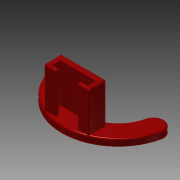
# Autodesk Inventor part: Camerahouder
Saved by Autodesk Inventor 2015 (Build 190159000, 159)
## iProperties
Created: 2016-04-29
Part Number: Camerahouder
Material: Generic
Document SubType Name: Modeling
Designer: david
Density: 1 g/cm^3
Appearance: Red
Author: david
Autodesk Inventor part; units mm, degrees
ref_plane "YZ Plane" through (0, 0, 0) normal (1, 0, 0) x (0, 1, 0)
ref_plane "XZ Plane" through (0, 0, 0) normal (0, 1, 0) x (-1, 0, 0)
ref_plane "XY Plane" through (0, 0, 0) normal (0, 0, 1) x (1, 0, 0)
sketch "Sketch1" plane through (0, 0, 0) normal (0, 0, 1) x (1, 0, 0)
  circle A0 centre (0, 0) radius 27.5
  circle A1 centre (0, 0) radius 42.5
  line L0 (27.5, 0) -> (42.5, 0)
  line L1 (-27.5, 0) -> (-42.5, 0)
  dimension "d0" = 55
  dimension "d1" = 85
  constraints: 4 end point, 4 point on circle, 2 centre point, 2 coincident, 2 point on line, 1 horizontal
  measures "d0" diameter of A0
  measures "d1" diameter of A1
extrude "Extrusion1" add sketch "Sketch1" along normal blind 5 contours L0 A1 L1 A0 picked at (1.1049, -37.278)
fillet "Fillet1" radius 7.5 4 edges at (-27.5, 0, 2.5) (-42.5, 0, 2.5) (27.5, 0, 2.5) (42.5, 0, 2.5)
sketch "Sketch2" plane through (0, 0, 5) normal (0, 0, 1) x (1, 0, 0)
  line L0 (15, -30) -> (-15, -30)
  line L1 (-15, -30) -> (-15, -38.9796)
  line L2 (-15, -38.9796) -> (15, -38.9796)
  line L3 (15, -38.9796) -> (15, -30)
  line L4 (15, -30) -> (-15, -38.9796) construction
  line L5 (-15, -30) -> (15, -38.9796) construction
  point P0 (0, 0)
  point P1 (0, -34.4898)
  dimension "d5" = 30
  dimension "d6" = 30
  constraints: 12 end point, 2 midpoint, 2 parallel, 1 horizontal, 1 perpendicular
  measures "d5" distance of L1.end L2.end
  measures "d6" distance from line of point (0, 0) L0
extrude "Extrusion2" add sketch "Sketch2" along normal blind 30
sketch "Sketch3" plane through (0, 0, 35) normal (0, 0, 1) x (1, 0, 0)
  line L0 (-8, -38.9796) -> (8, -38.9796)
  line L1 (8, -38.9796) -> (8, -35.9796)
  line L2 (8, -35.9796) -> (-8, -35.9796)
  line L3 (-8, -35.9796) -> (-8, -38.9796)
  line L4 (-8, -38.9796) -> (8, -35.9796) construction
  line L5 (8, -38.9796) -> (-8, -35.9796) construction
  line L6 (-15, -38.9796) -> (15, -38.9796) projected
  line L7 (-13, -27.9796) -> (13, -27.9796)
  line L8 (13, -27.9796) -> (13, -35.9796)
  line L9 (13, -35.9796) -> (-13, -35.9796)
  line L10 (-13, -35.9796) -> (-13, -27.9796)
  line L11 (-13, -27.9796) -> (13, -35.9796) construction
  line L12 (13, -27.9796) -> (-13, -35.9796) construction
  point P0 (0, 0)
  point P1 (0, -37.4796)
  point P2 (0, -31.9796)
  dimension "d9" = 16
  dimension "d10" = 3
  dimension "d11" = 0
  dimension "d12" = 26
  dimension "d24" = 8
  constraints: 24 end point, 4 midpoint, 4 parallel, 2 horizontal, 2 perpendicular
  measures "d9" distance of L2.end L1.end
  measures "d10" distance of L2.end L0.start
  measures "d11" distance from line of L6 L0.start
  measures "d12" distance of L8.end L9.end
  measures "d24" distance between parallel lines of L7 L2
extrude "Extrusion3" cut sketch "Sketch3" against normal blind 30
sketch "Sketch4" plane through (-15, -30, 5) normal (0, 1, 0) x (1, 0, 0)
  line L0 (-26.5128, 0) -> (56.5128, 0) projected
  line L1 (30, -30) -> (0, -30)
  line L2 (0, -30) -> (0, 0)
  line L3 (0, 0) -> (30, 0)
  line L4 (30, 0) -> (30, -30)
  line L5 (30, 0) -> (0, 0)
  line L6 (0, 0) -> (0, 5)
  line L7 (0, 5) -> (30, 5)
  line L8 (30, 5) -> (30, 0)
  point P0 (15, 5)
  dimension "d15" = 30
  dimension "d18" = 30
  dimension "d19" = 5
  constraints: 16 end point, 4 parallel, 2 horizontal, 2 perpendicular, 1 point on line
  measures "d15" distance of L2.end L3.end
  measures "d18" distance of L6.end L7.end
  measures "d19" distance between parallel lines of L0 L7
extrude "Extrusion4" add sketch "Sketch4" along normal blind 4 contours L0 L4 L1 L2
sketch "Sketch5" plane through (-15, -38.9796, 5) normal (-1, 0, 0) x (0, 0, 1)
  line L0 (30, 12.9796) -> (0, 12.9796)
  line L1 (0, 12.9796) -> (0, 0)
  line L2 (0, 0) -> (30, 0)
  line L3 (30, 0) -> (30, 12.9796)
  point P0 (-5, 38.9796)
  constraints: 8 end point, 2 parallel, 1 horizontal, 1 perpendicular
extrude "Extrusion5" add sketch "Sketch5" along normal blind 2
sketch "Sketch6" plane through (15, -38.9796, 35) normal (1, 0, 0) x (0, 0, -1)
  line L0 (0, 0) -> (30, 0)
  line L1 (30, 0) -> (30, 12.9796)
  line L2 (30, 12.9796) -> (0, 12.9796)
  line L3 (0, 12.9796) -> (0, 0)
  point P0 (35, 38.9796)
  constraints: 8 end point, 2 parallel, 1 horizontal, 1 perpendicular
extrude "Extrusion6" add sketch "Sketch6" along normal blind 2
fillet "Fillet2" radius 1 10 edges at (17, -38.9796, 20) (8, -38.9796, 20) (-8, -38.9796, 20) (-8, -35.9796, 20) (-17, -38.9796, 20) (17, -26, 20) (-17, -26, 20) (-17, -32.4898, 35) (-12.5, -38.9796, 35) (-13, -32.9898, 35)
fillet "Fillet3" radius 1 25 edges at (-16.7071, -26.2929, 34.7071) (16.7071, -26.2929, 35) (17, -32.4898, 35) (16.7071, -38.6867, 35) (12.5, -38.9796, 35) (8.2929, -38.6867, 35) (8, -36.9796, 35) (0, -26, 35) (-0.5, -30, 35) (10.5, -35.9796, 35) (13, -32.9898, 35) (-8, -37.4796, 35) (-8.2929, -38.6867, 34.7071) (-11.5, -35.9796, 35) (-8.2929, -36.2725, 35) (0, -26, 5) (-29.4861, -1.656, 5) (-34.187, 0, 5) (-40.031, -2.7991, 5) (0, -42.5, 5) (40.031, -2.7991, 5) (34.187, 0, 5) (29.4861, -1.656, 5) (20.5386, -18.2871, 5) (-20.5386, -18.2871, 5)
body "Solid1"
